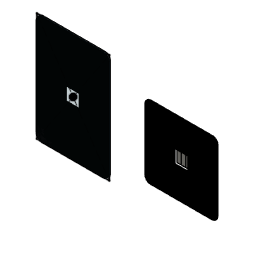
Acrylic Plates & Foam v4 (LEDs 3 strips of 5) (Autodesk Fusion 360 design; units mm, degrees)
Autodesk Fusion 360 part; units mm, degrees
sketch "Sketch1" plane through (0, 0, 0) normal (0, 1, 0) x (1, 0, 0)
  line L0 (100, -100) -> (-100, -100)
  line L1 (-100, -100) -> (-100, 100)
  line L2 (-100, 100) -> (100, 100)
  line L3 (100, 100) -> (100, -100)
  line L4 (100, -100) -> (-100, 100) construction
  line L5 (-100, -100) -> (100, 100) construction
  dimension "d1" = 200
  dimension "d2" = 200
  constraint horizontal L0
  constraint perpendicular L0 L1
  constraint parallel L0 L2
  constraint parallel L1 L3
  constraint coincident L4 origin
  constraint coincident L5 origin
  measures "d1" distance of L1.end L2.end
  measures "d2" distance of L0.end L1.end
extrude "Extrude1" add sketch "Sketch1" along normal blind 3 makes body 1
fillet "Fillet1" radius 15 4 edges at (100, 1.5, 100) (-100, 1.5, 100) (100, 1.5, -100) (-100, 1.5, -100) on bodies 1
sketch "Sketch2" plane through (0, 0, 0) normal (0, -1, 0) x (1, 0, 0)
  arc A0 (-100, -85) -> (-85, -100) centre (-85, -85) ccw
  line L0 (-85, -100) -> (85, -100)
  arc A1 (85, -100) -> (100, -85) centre (85, -85) ccw
  line L1 (100, -85) -> (100, 85)
  arc A2 (100, 85) -> (85, 100) centre (85, 85) ccw
  line L2 (85, 100) -> (-85, 100)
  arc A3 (-85, 100) -> (-100, 85) centre (-85, 85) ccw
  line L3 (-100, 85) -> (-100, -85)
  line L4 (0, 0) -> (0, 50) construction
  line L5 (25.5, 56.5) -> (-25.5, 56.5)
  line L6 (-25.5, 56.5) -> (-25.5, 43.5)
  line L7 (-25.5, 43.5) -> (25.5, 43.5)
  line L8 (25.5, 43.5) -> (25.5, 56.5)
  line L9 (25.5, 56.5) -> (-25.5, 43.5) construction
  line L10 (-25.5, 56.5) -> (25.5, 43.5) construction
  line L11 (0, 0) -> (29, 0) construction
  line L12 (-25.5, -56.5) -> (25.5, -43.5) construction
  line L13 (25.5, -56.5) -> (-25.5, -56.5)
  line L14 (-25.5, -43.5) -> (25.5, -43.5)
  line L15 (25.5, -56.5) -> (-25.5, -43.5) construction
  line L16 (-25.5, -56.5) -> (-25.5, -43.5)
  line L17 (25.5, -43.5) -> (25.5, -56.5)
  point P0 (0, 50)
  point P1 (0, -50)
  point P2 (0, -50)
  dimension "d7" = 50
  dimension "d9" = 51
  dimension "d10" = 13
  constraint vertical L4
  constraint coincident L4.start L11.start
  constraint horizontal L5
  constraint perpendicular L5 L6
  constraint parallel L5 L7
  constraint parallel L6 L8
  constraint coincident L9 P0
  constraint coincident L10 P0
  constraint coincident P0 L4.end
  constraint perpendicular L4 L11
  constraint symmetric P0 L11 P2
  constraint symmetric L5.start L11 L13.start
  constraint symmetric L5.end L11 L12.start
  constraint symmetric L6.end L11 L14.start
  constraint symmetric L7.end L11 L12.end
  measures "d7" distance of L4.start P0
  measures "d9" distance of L6.end L7.end
  measures "d10" distance of L5.end L6.end
extrude "Extrude1'" add sketch "Sketch2" along normal blind 2 separate body makes body 2 in component "Foam Protector"
copy_body "Body->Comp1" bodies 1 removing the originals makes body 3 in component "Acrylic sheet"
sketch "Sketch1 (2)" plane through (0, 0, 0) normal (0, 1, 0) x (1, 0, 0) in component "Acrylic sheet"
  line L0 (100, -150) -> (-100, -150)
  line L1 (-100, -150) -> (-100, 150)
  line L2 (-100, 150) -> (100, 150)
  line L3 (100, 150) -> (100, -150)
  line L4 (100, -150) -> (-100, 150) construction
  line L5 (-100, -150) -> (100, 150) construction
  dimension "d15" = 200
  dimension "d16" = 300
  constraint horizontal L0
  constraint perpendicular L0 L1
  constraint parallel L0 L2
  constraint parallel L1 L3
  constraint coincident L4 origin
  constraint coincident L5 origin
  measures "d15" distance of L1.end L2.end
  measures "d16" distance of L0.end L1.end
extrude "Extrude1''" add sketch "Sketch1 (2)" along normal blind 3 separate body makes body 4 in component "Acrylic sheet"
fillet "Fillet1'" radius 15 4 edges at (100, 1.5, 150) (-100, 1.5, 150) (100, 1.5, -150) (-100, 1.5, -150) on bodies 4 in component "Acrylic sheet"
sketch "Sketch1 (3)" plane through (0, 0, 0) normal (0, -1, 0) x (1, 0, 0) in component "Foam Protector"
  arc A0 (-100, -135) -> (-85, -150) centre (-85, -135) ccw
  line L0 (-85, -150) -> (85, -150)
  arc A1 (85, -150) -> (100, -135) centre (85, -135) ccw
  line L1 (100, -135) -> (100, 135)
  arc A2 (100, 135) -> (85, 150) centre (85, 135) ccw
  line L2 (85, 150) -> (-85, 150)
  arc A3 (-85, 150) -> (-100, 135) centre (-85, 135) ccw
  line L3 (-100, 135) -> (-100, -135)
  line L4 (0, 0) -> (0, 50) construction
  line L5 (0, 0) -> (15, 0) construction
  line L6 (25.5, 56.5) -> (-25.5, 56.5)
  line L7 (-25.5, 56.5) -> (-25.5, 43.5)
  line L8 (-25.5, 43.5) -> (25.5, 43.5)
  line L9 (25.5, 43.5) -> (25.5, 56.5)
  line L10 (25.5, 56.5) -> (-25.5, 43.5) construction
  line L11 (-25.5, 56.5) -> (25.5, 43.5) construction
  line L12 (-25.5, -56.5) -> (25.5, -43.5) construction
  line L13 (25.5, -56.5) -> (-25.5, -43.5) construction
  line L14 (25.5, -43.5) -> (25.5, -56.5)
  line L15 (-25.5, -56.5) -> (-25.5, -43.5)
  line L16 (-25.5, -43.5) -> (25.5, -43.5)
  line L17 (25.5, -56.5) -> (-25.5, -56.5)
  point P0 (0, 50)
  point P1 (0, -50)
  point P2 (0, -50)
  dimension "d21" = 50
  dimension "d22" = 51
  dimension "d23" = 13
  constraint vertical L4
  constraint coincident L4.start L5.start
  constraint perpendicular L4 L5
  constraint horizontal L6
  constraint perpendicular L6 L7
  constraint parallel L6 L8
  constraint parallel L7 L9
  constraint coincident L10 P0
  constraint coincident L11 P0
  constraint coincident P0 L4.end
  constraint symmetric P0 L5 P2
  constraint symmetric L5 L6.start L13.start
  constraint symmetric L5 L6.end L12.start
  constraint symmetric L5 L7.end L13.end
  constraint symmetric L5 L8.end L12.end
  constraint symmetric L5 P0 P2
  measures "d21" distance of L4.start P0
  measures "d22" distance of L7.end L8.end
  measures "d23" distance of L6.end L7.end
extrude "Extrude2" add sketch "Sketch1 (3)" along normal blind 2 separate body makes body 5 in component "Foam Protector"
fillet "Fillet1''" radius 2.5 4 edges at (-25.5, -1, 43.5) (-25.5, -1, 56.5) (25.5, -1, 43.5) (25.5, -1, 56.5) on bodies 5 in component "Foam Protector"
fillet "Fillet1''" radius 2.5 4 edges at (25.5, -1, -43.5) (25.5, -1, -56.5) (-25.5, -1, -43.5) (-25.5, -1, -56.5) on bodies 5 in component "Foam Protector"
fillet "Fillet2" radius 2.5 4 edges at (-25.5, -1, -56.5) (-25.5, -1, -43.5) (25.5, -1, -56.5) (25.5, -1, -43.5) on bodies 2 in component "Foam Protector"
move_body "Move1" bodies 3 to x (1, 0, 0) y (0, 1, 0) z (0, 0, 1) at (300, 0, 0) in component "Acrylic sheet"
move_body "Move1'" bodies 2 to x (1, 0, 0) y (0, 1, 0) z (0, 0, 1) at (300, 0, 0) in component "Foam Protector"
sketch "Sketch2 (2)" plane through (0, 0, 0) normal (0, -1, 0) x (1, 0, 0) in component "Foam Protector"
  arc A0 (200, -85) -> (215, -100) centre (215, -85) ccw
  line L0 (215, -100) -> (385, -100)
  arc A1 (385, -100) -> (400, -85) centre (385, -85) ccw
  line L1 (400, -85) -> (400, 85)
  arc A2 (400, 85) -> (385, 100) centre (385, 85) ccw
  line L2 (385, 100) -> (215, 100)
  arc A3 (215, 100) -> (200, 85) centre (215, 85) ccw
  line L3 (200, 85) -> (200, -85)
  line L4 (300, 100) -> (300, 0) construction
  line L5 (315.5, 18.5) -> (284.5, 18.5)
  line L6 (284.5, 18.5) -> (284.5, -18.5)
  line L7 (284.5, -18.5) -> (315.5, -18.5)
  line L8 (315.5, -18.5) -> (315.5, 18.5)
  line L9 (315.5, 18.5) -> (284.5, -18.5) construction
  line L10 (284.5, 18.5) -> (315.5, -18.5) construction
  point P0 (300, 0)
  dimension "d32" = 31
  dimension "d33" = 37
  constraint midpoint L2 L4.start
  constraint perpendicular L2 L4
  constraint horizontal L5
  constraint perpendicular L5 L6
  constraint parallel L5 L7
  constraint parallel L6 L8
  constraint coincident L9 P0
  constraint coincident L10 P0
  constraint coincident P0 L4.end
  measures "d32" distance of L6.end L7.end
  measures "d33" distance of L5.end L6.end
extrude "Extrude3" add sketch "Sketch2 (2)" along normal blind 2 separate body makes body 6 in component "Foam Protector"
sketch "Sketch3" plane through (0, 0, 0) normal (0, -1, 0) x (1, 0, 0) in component "Foam Protector"
  arc A0 (200, -85) -> (215, -100) centre (215, -85) ccw
  line L0 (215, -100) -> (385, -100)
  arc A1 (385, -100) -> (400, -85) centre (385, -85) ccw
  line L1 (400, -85) -> (400, 85)
  arc A2 (400, 85) -> (385, 100) centre (385, 85) ccw
  line L2 (385, 100) -> (215, 100)
  arc A3 (215, 100) -> (200, 85) centre (215, 85) ccw
  line L3 (200, 85) -> (200, -85)
  line L4 (300, 100) -> (300, 0) construction
  line L5 (318.75, 18.5) -> (281.25, 18.5)
  line L6 (281.25, 18.5) -> (281.25, -18.5)
  line L7 (281.25, -18.5) -> (318.75, -18.5)
  line L8 (318.75, -18.5) -> (318.75, 18.5)
  line L9 (318.75, 18.5) -> (281.25, -18.5) construction
  line L10 (281.25, 18.5) -> (318.75, -18.5) construction
  point P0 (300, 0)
  dimension "d36" = 100
  dimension "d37" = 37.5
  dimension "d38" = 37
  constraint vertical L4
  constraint midpoint L2 L4.start
  constraint horizontal L5
  constraint perpendicular L5 L6
  constraint parallel L5 L7
  constraint parallel L6 L8
  constraint coincident L9 P0
  constraint coincident L10 P0
  constraint coincident P0 L4.end
  measures "d36" distance of L4.start P0
  measures "d37" distance of L6.end L7.end
  measures "d38" distance of L5.end L6.end
extrude "Extrude4" add sketch "Sketch3" along normal blind 2 separate body makes body 7 in component "Foam Protector"
move_body "Move2" bodies 6 to x (1, 0, 0) y (0, 1, 0) z (0, 0, 1) at (0, 0, 250) in component "Foam Protector"
move_body "Move3" bodies 7 to x (1, 0, 0) y (0, 1, 0) z (0, 0, 1) at (0, 0, 500) in component "Foam Protector"
sketch "Sketch4" plane through (0, 0, 0) normal (0, -1, 0) x (1, 0, 0) in component "Foam Protector"
  arc A0 (-100, -135) -> (-85, -150) centre (-85, -135) ccw
  line L0 (-85, -150) -> (85, -150)
  arc A1 (85, -150) -> (100, -135) centre (85, -135) ccw
  line L1 (100, -135) -> (100, 135)
  arc A2 (100, 135) -> (85, 150) centre (85, 135) ccw
  line L2 (85, 150) -> (-85, 150)
  arc A3 (-85, 150) -> (-100, 135) centre (-85, 135) ccw
  line L3 (-100, 135) -> (-100, -135)
  line L4 (18.5, 18.75) -> (-18.5, 18.75)
  line L5 (-18.5, 18.75) -> (-18.5, -18.75)
  line L6 (-18.5, -18.75) -> (18.5, -18.75)
  line L7 (18.5, -18.75) -> (18.5, 18.75)
  line L8 (18.5, 18.75) -> (-18.5, -18.75) construction
  line L9 (-18.5, 18.75) -> (18.5, -18.75) construction
  dimension "d41" = 37
  dimension "d42" = 37.5
  constraint horizontal L4
  constraint perpendicular L4 L5
  constraint parallel L4 L6
  constraint parallel L5 L7
  constraint coincident L8 origin
  constraint coincident L9 origin
  measures "d41" distance of L5.end L6.end
  measures "d42" distance of L4.end L5.end
extrude "Extrude5" add sketch "Sketch4" along normal blind 2 separate body makes body 8 in component "Foam Protector"
sketch "Sketch5" plane through (0, 0, 0) normal (0, -1, 0) x (1, 0, 0) in component "Foam Protector"
  arc A0 (200, -85) -> (215, -100) centre (215, -85) ccw
  line L0 (215, -100) -> (385, -100)
  arc A1 (385, -100) -> (400, -85) centre (385, -85) ccw
  line L1 (400, -85) -> (400, 85)
  arc A2 (400, 85) -> (385, 100) centre (385, 85) ccw
  line L2 (385, 100) -> (215, 100)
  arc A3 (215, 100) -> (200, 85) centre (215, 85) ccw
  line L3 (200, 85) -> (200, -85)
  line L4 (318.5, 18.75) -> (281.5, 18.75)
  line L5 (281.5, 18.75) -> (281.5, -18.75)
  line L6 (281.5, -18.75) -> (318.5, -18.75)
  line L7 (318.5, -18.75) -> (318.5, 18.75)
  line L8 (318.5, 18.75) -> (281.5, -18.75) construction
  line L9 (281.5, 18.75) -> (318.5, -18.75) construction
  point P0 (300, 0)
  dimension "d45" = 37
  dimension "d46" = 37.5
  constraint horizontal L4
  constraint perpendicular L4 L5
  constraint parallel L4 L6
  constraint parallel L5 L7
  constraint coincident L8 P0
  constraint coincident L9 P0
  measures "d45" distance of L5.end L6.end
  measures "d46" distance of L4.end L5.end
extrude "Extrude6" add sketch "Sketch5" along normal blind 2 separate body makes body 9 in component "Foam Protector"
fillet "Fillet3" radius 2 8 edges at (18.5, -1, 18.75) (18.5, -1, -18.75) (-18.5, -1, 18.75) (-18.5, -1, -18.75) (281.5, -1, -18.75) (281.5, -1, 18.75) (318.5, -1, -18.75) (318.5, -1, 18.75) on bodies 8 9 in component "Foam Protector"
sketch "Sketch3 (2)" plane through (0, 3, 0) normal (0, 1, 0) x (-1, 0, 0)
  arc A0 (-215, -100) -> (-200, -85) centre (-215, -85) ccw
  line L0 (-200, -85) -> (-200, 85)
  arc A1 (-200, 85) -> (-215, 100) centre (-215, 85) ccw
  line L1 (-215, 100) -> (-385, 100)
  arc A2 (-385, 100) -> (-400, 85) centre (-385, 85) ccw
  line L2 (-400, 85) -> (-400, -85)
  arc A3 (-400, -85) -> (-385, -100) centre (-385, -85) ccw
  line L3 (-385, -100) -> (-215, -100)
  line L4 (-294, 18.25) -> (-306, 18.25)
  line L5 (-306, 18.25) -> (-306, -18.25)
  line L6 (-306, -18.25) -> (-294, -18.25)
  line L7 (-294, -18.25) -> (-294, 18.25)
  line L8 (-294, 18.25) -> (-306, -18.25) construction
  line L9 (-306, 18.25) -> (-294, -18.25) construction
  line L10 (-297.525, 2.475) -> (-302.475, 2.475)
  line L11 (-302.475, 2.475) -> (-302.475, -2.475)
  line L12 (-302.475, -2.475) -> (-297.525, -2.475)
  line L13 (-297.525, -2.475) -> (-297.525, 2.475)
  line L14 (-297.525, 2.475) -> (-302.475, -2.475) construction
  line L15 (-302.475, 2.475) -> (-297.525, -2.475) construction
  circle A4 centre (-300, 0) radius 1.75
  line L16 (-297.525, 9.475) -> (-302.475, 4.525) construction
  line L17 (-297.525, 9.475) -> (-302.475, 9.475)
  line L18 (-297.525, 4.525) -> (-297.525, 9.475)
  line L19 (-302.475, 9.475) -> (-297.525, 4.525) construction
  line L20 (-302.475, 4.525) -> (-297.525, 4.525)
  circle A5 centre (-300, 7) radius 1.75
  line L21 (-302.475, 9.475) -> (-302.475, 4.525)
  line L22 (-297.525, 16.475) -> (-302.475, 11.525) construction
  line L23 (-297.525, 16.475) -> (-302.475, 16.475)
  line L24 (-297.525, 11.525) -> (-297.525, 16.475)
  line L25 (-302.475, 16.475) -> (-297.525, 11.525) construction
  line L26 (-302.475, 11.525) -> (-297.525, 11.525)
  circle A6 centre (-300, 14) radius 1.75
  line L27 (-302.475, 16.475) -> (-302.475, 11.525)
  line L28 (-297.525, -4.525) -> (-302.475, -4.525)
  line L29 (-302.475, -9.475) -> (-297.525, -9.475)
  line L30 (-302.475, -4.525) -> (-297.525, -9.475) construction
  circle A7 centre (-300, -7) radius 1.75
  line L31 (-302.475, -4.525) -> (-302.475, -9.475)
  line L32 (-297.525, -9.475) -> (-297.525, -4.525)
  line L33 (-297.525, -4.525) -> (-302.475, -9.475) construction
  line L34 (-297.525, -11.525) -> (-302.475, -11.525)
  line L35 (-302.475, -16.475) -> (-297.525, -16.475)
  line L36 (-302.475, -11.525) -> (-297.525, -16.475) construction
  circle A8 centre (-300, -14) radius 1.75
  line L37 (-302.475, -11.525) -> (-302.475, -16.475)
  line L38 (-297.525, -16.475) -> (-297.525, -11.525)
  line L39 (-297.525, -11.525) -> (-302.475, -16.475) construction
  point P0 (-300, 0)
  point P1 (-300, 0)
  point P2 (-300, 7)
  point P3 (-300, 7)
  point P4 (-300, 14)
  point P5 (-300, 14)
  point P6 (-300, -7)
  point P7 (-300, -7)
  point P8 (-300, -14)
  point P9 (-300, -14)
  dimension "d51" = 12
  dimension "d52" = 36.5
  dimension "d53" = 4.95
  dimension "d54" = 4.95
  dimension "d55" = 3.5
  dimension "d66" = 0
  dimension "d67" = 14
  dimension "d70" = 0
  dimension "d71" = -14
  constraint horizontal L4
  constraint perpendicular L4 L5
  constraint parallel L4 L6
  constraint parallel L5 L7
  constraint coincident L8 P1
  constraint coincident L9 P1
  constraint horizontal L10
  constraint perpendicular L10 L11
  constraint parallel L10 L12
  constraint parallel L11 L13
  constraint coincident L14 P1
  constraint coincident L15 P1
  constraint coincident P1 P0
  measures "d51" distance of L5.end L6.end
  measures "d52" distance of L4.end L5.end
  measures "d53" distance of L11.end L12.end
  measures "d54" distance of L10.end L11.end
  measures "d55" diameter of A4
extrude "Extrude1'''" add sketch "Sketch3 (2)" along normal blind 2 separate body contours L4 L5 L6 L7 | L10 L11 L12 L13 | A4 | L17 L18 L20 L21 | A5 | L23 L24 L26 L27 | A6 | L28 L29 L31 L32 | A7 | L34 L35 L37 L38 | A8 makes body 10 in component "LEDs"
extrude "Extrude2'" cut sketch "Sketch3 (2)" along normal blind 1.5 contours L4 L5 L6 L7 bodies 10 in component "LEDs"
extrude "Extrude3'" cut sketch "Sketch3 (2)" along normal blind 0.5 contours A4 | A5 | A6 | A7 | A8 bodies 10 in component "LEDs"
pattern_linear "R-Pattern1" count 2 spacing 12.25 along (1, 0, 0) of bodies 10 makes body 11 in component "LEDs"
pattern_linear "R-Pattern2" count 2 spacing 12.25 along (-1, 0, 0) of bodies 10 makes body 12 in component "LEDs"
split "Split1" by plane through (12.25, 4.5, 0) normal (0, -1, 0) bodies 12 10 11 makes body 23 at (312.2936, 3, 11.7683) makes body 24 at (312.2936, 3, 4.7683) makes body 25 at (312.2936, 3, -2.2317) makes body 26 at (312.2936, 3, -11.7683) makes body 27 at (312.2936, 3, -9.2317) makes body 18 at (300.0436, 3, 11.7683) makes body 19 at (300.0436, 3, 4.7683) makes body 20 at (300.0436, 3, -2.2317) makes body 21 at (300.0436, 3, -11.7683) makes body 22 at (300.0436, 3, -9.2317) makes body 13 at (287.7936, 3, 11.7683) makes body 14 at (287.7936, 3, 4.7683) makes body 15 at (287.7936, 3, -2.2317) makes body 16 at (287.7936, 3, -11.7683) makes body 17 at (287.7936, 3, -9.2317) in component "LEDs"
component "Foam Protector" placed x (1, 0, 0) y (0, 1, 0) z (0, 0, 1) at (0, 0, 0)
component "Acrylic sheet" placed x (1, 0, 0) y (0, 1, 0) z (0, 0, 1) at (0, 0, 0)
component "LEDs" placed x (1, 0, 0) y (0, 1, 0) z (0, 0, 1) at (0, 0, 0)
hidden bodies 2 5 6 7 3
equation "d32 = 30 mm + 1 mm"
equation "d33 = ( 12 * 3 ) * 1 mm + 1 mm"
equation "d37 = 36.5 mm + 1 mm"
equation "d38 = ( 12 * 3 ) * 1 mm + 1 mm"
equation "d41 = ( 12 * 3 ) * 1 mm + 1 mm"
equation "d42 = 36.5 mm + 1 mm"
equation "d45 = ( 12 * 3 ) * 1 mm + 1 mm"
equation "d46 = 36.5 mm + 1 mm"
named bodies: "(Decided against) 200x200 - Double 1x7", "200x200", "200x300", "(Decided against) 200x300 - Double 1x7", "(Decided against) 200x200 - Single 3x4", "(Decided against) 200x200-Single 3x5", "200x300 - LED Grid 5x3", "200x200 - LED Grid 5x3"
